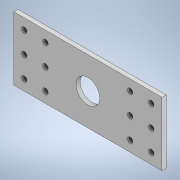
# Autodesk Inventor part: Bearing Plate Long
Saved by Autodesk Inventor 2020 (Build 240168000, 168)
## iProperties
Created: 2020-02-11
Part Number: Bearing Plate Long
Material: Generic
Document SubType Name: Modeling
Designer: 339294
Density: 1 g/cm^3
Appearance: Default
Author: 339294
Autodesk Inventor part; units mm, degrees
ref_plane "YZ Plane" through (0, 0, 0) normal (1, 0, 0) x (0, 1, 0)
ref_plane "XZ Plane" through (0, 0, 0) normal (0, 1, 0) x (-1, 0, 0)
ref_plane "XY Plane" through (0, 0, 0) normal (0, 0, 1) x (1, 0, 0)
sketch "Sketch1" plane through (0, 0, 0) normal (0, 0, 1) x (1, 0, 0)
  line L0 (0, 0) -> (177.8, 0)
  line L1 (177.8, 0) -> (177.8, 76.2)
  line L2 (177.8, 76.2) -> (0, 76.2)
  line L3 (0, 76.2) -> (0, 0)
  circle A0 centre (88.9, 38.1) radius 14.2875
  circle A1 centre (12.7, 63.5) radius 3.2512
  circle A2 centre (38.1, 63.5) radius 3.2512
  circle A3 centre (12.7, 38.1) radius 3.2512
  circle A4 centre (38.1, 38.1) radius 3.2512
  circle A5 centre (12.7, 12.7) radius 3.2512
  circle A6 centre (38.1, 12.7) radius 3.2512
  circle A7 centre (139.7, 63.5) radius 3.2512
  circle A8 centre (165.1, 63.5) radius 3.2512
  circle A9 centre (139.7, 38.1) radius 3.2512
  circle A10 centre (165.1, 38.1) radius 3.2512
  circle A11 centre (139.7, 12.7) radius 3.2512
  circle A12 centre (165.1, 12.7) radius 3.2512
  dimension "d0" = 177.8
  dimension "d1" = 76.2
  dimension "d2" = 38.1
  dimension "d3" = 88.9
  dimension "d4" = 28.575
  dimension "d5" = 6.5024
  dimension "d6" = 12.7
  dimension "d7" = 12.7
  dimension "d10" = 25.4
  dimension "d13" = 25.4
  dimension "d20" = 127
  constraints: 13 centre point, 8 end point, 3 horizontal, 2 parallel, 1 perpendicular, 1 vertical, 22 other
  measures "d0" distance of L2.end L1.end
  measures "d1" distance of L1.end L0.end
  measures "d2" distance from line of L2 A0.centre
  measures "d3" distance from line of L1 A0.centre
  measures "d4" diameter of A0
  measures "d5" diameter of A1
  measures "d6" distance from line of L2 A1.centre
  measures "d7" distance from line of L3 A1.centre
  measures "d10" distance of A1.centre A2.centre
  measures "d13" distance of A1.centre A3.centre
  measures "d20" distance of A1.centre A7.centre
extrude "Extrusion2" add sketch "Sketch1" along normal blind 5.08
equation "\"d2\" = 0.5 * d1"
body "Solid2"
